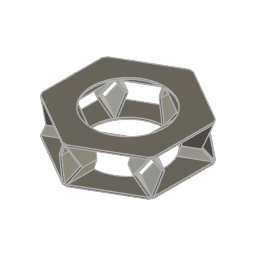
Parametric TPU Printable Horn Ring Support (Autodesk Fusion 360 design; units mm, degrees)
Autodesk Fusion 360 part; units mm, degrees
sketch "Sketch1" plane through (0, 0, 0) normal (1, 0, 0) x (0, 1, 0) in component "Component"
  line L0 (0, 0) -> (35, 0)
  line L1 (35, 9) -> (20, 9)
  line L2 (35, 9) -> (35, 10)
  line L3 (35, 10) -> (20, 10)
  line L4 (20, 10) -> (20, 9)
  line L5 (20, 9) -> (23.5, 0)
  line L6 (35, 9) -> (31.5, 0)
  line L7 (23.5, 0) -> (31.5, 0)
  line L8 (35, 9) -> (35, 0)
  line L9 (20, 9) -> (20, 0)
  dimension "d27" = 35
  dimension "d28" = 20
  dimension "d29" = 1
  dimension "d30" = 10
  dimension "d34" = 8
  constraint coincident L0.start origin
  constraint horizontal L0
  constraint horizontal L1
  constraint perpendicular L1 L2
  constraint perpendicular L2 L3
  constraint perpendicular L3 L4
  constraint coincident L0 L5.end
  constraint coincident L0 L6.end
  constraint equal L5 L6
  constraint perpendicular L0 L8
  constraint coincident L0 L9.end
  constraint perpendicular L0 L9
  measures "d27" horizontal distance of L0.start L2.end
  measures "d28" horizontal distance of L0.start L3.end
  measures "d29" distance of L1.end L3.end
  measures "d30" vertical distance of L0.start L3.end
  measures "d34" distance of L5.end L6.end
sketch "Sketch2" plane through (0, 0, 0) normal (0, 1, 0) x (1, 0, 0) in component "Component"
  line L0 (0, -9) -> (5.1962, 0)
  line L1 (5.1962, 0) -> (6.3962, 0)
  line L2 (6.3962, 0) -> (1.2, -9)
  line L3 (1.2, -9) -> (0, -9)
  line L4 (0, 0) -> (0, -9) construction
  line L5 (0, 0) -> (0, -9) construction
  line L6 (-6.3962, 0) -> (-1.2, -9)
  line L7 (-5.1962, 0) -> (-6.3962, 0)
  line L8 (0, -9) -> (-5.1962, 0)
  line L9 (-1.2, -9) -> (0, -9)
  point P0 (0, -9)
  dimension "d35" = 1.2
  dimension "d36" = 60
  constraint coincident P0 L0.start
  constraint horizontal L1
  constraint parallel L0 L2
  constraint horizontal L3
  constraint coincident L4.start L5.start
  constraint symmetric P0 L4 L0.start
  constraint symmetric L0.end L4 L7.start
  constraint symmetric L1.end L4 L6.start
  constraint symmetric L2.end L4 L6.end
  constraint symmetric L5.start L4 origin
  constraint coincident L1 L4.start
  measures "d35" distance of L0.end L1.end
  measures "d36" angle of L0 L8
extrude "Extrude1" add sketch "Sketch2" along normal blind 15 from surface at 20 makes body 1 in component "Component"
extrude "Extrude2" cut sketch "Sketch1" along normal through all and the other way through all contours L0 L5 L9 | L0 L6 L8 bodies 1 in component "Component"
revolve "Revolve1" add sketch "Sketch1" angle 360 about axis through (0, 0, 1.75) along (0, 0, 1) separate body contours L1 L2 L3 L4 makes body 2 in component "Component"
sketch "Sketch3" plane through (0, 0, 10) normal (0, 0, 1) x (-1, 0, 0) in component "Component"
  circle A0 centre (0, 0) radius 20
  circle A1 centre (0, 0) radius 35
  line L0 (0, -35) -> (0, 0) construction
  circle A2 centre (0, 0) radius 20
  circle A3 centre (0, 0) radius 35
  line L1 (-1.2, -20) -> (-1.2, -35)
  line L2 (0, 0) -> (-30.3109, -17.5) construction
  line L3 (-29.6932, -18.5288) -> (-16.6894, -11.0211)
  line L4 (-16.6894, -11.0211) -> (-1.2, -20)
  line L5 (-29.6932, -18.5288) -> (-1.2, -35)
  point P0 (-1.2, -35)
  point P1 (0, -35)
  dimension "d56" = 60
  dimension "d57" = 1.2
  dimension "d58" = 1.2
  constraint coincident P1 L0.start
  constraint coincident A0.centre A1.centre
  constraint coincident A3 L2.end
  constraint coincident A3 L3.start
  constraint coincident A2 L3.end
  constraint parallel L2 L3
  constraint coincident L1.start L4.end
  constraint coincident P0 L1.end
  measures "d56" angle of L0 L2
  measures "d57" distance of P0 P1
  measures "d58" distance of L2.end L3.start
extrude "Extrude4" cut sketch "Sketch3" against normal up to surface (1 mm away) contours A1 A3 L5 bodies 2 in component "Component"
pattern_circular "C-Pattern2" count 6 over 360 about axis through (0, 0, 1.75) along (0, 0, 1) of "Extrude4" in component "Component"
pattern_circular "C-Pattern1" count 6 over 360 about axis through (0, 0, 1.75) along (0, 0, 1) of bodies 1 makes body 3 at (-21.195, 15.6226, 6) makes body 4 at (-24.127, -10.5441, 6) makes body 5 at (-2.9321, -26.1667, 6) makes body 6 at (26.4364, -11.8774, 6) makes body 7 at (21.195, 15.6226, 6) in component "Component"
combine "Combine1" operation add target body 1 tool bodies 7 6 5 3 4 2 in component "Component"
mirror "Mirror2" about plane through (0, 0, 0) normal (0, 0, 1) of bodies 1 merged in component "Component"
extrude "Extrude5" add sketch "Sketch3" along normal blind 0.2 from surface at -1 contours A0 A2 L4 picked at (-11.0178, -14.7006) bodies 1 in component "Component"
pattern_circular "C-Pattern4" count 6 over 360 about axis through (0, 0, 1.75) along (0, 0, 1) of "Extrude5" in component "Component"
component "Component" placed x (1, 0, 0) y (0, 1, 0) z (0, 0, 1) at (0, 0, 0)
equation "BearingOD = 70 mm"
equation "BearingID = 40 mm"
equation "BearingHeight = 20 mm"
equation "TopBottomThickness = 1 mm"
equation "SupportCount = 6"
equation "d27 = BearingOD / 2"
equation "d28 = BearingID / 2"
equation "d29 = TopBottomThickness"
equation "d30 = BearingHeight / 2"
equation "d35 = WallThickness"
equation "d37 = BearingID / 2"
equation "d38 = ( BearingOD - BearingID ) / 2"
equation "d42 = SupportCount"
equation "NozzleSize = 0.4 mm"
equation "WallThickness = 3 * NozzleSize"
equation "d56 = ( 360 / SupportCount ) * 1 deg"
equation "d58 = d57"
equation "LayerHeightForBridgyBit = 0.2 mm"
equation "d63 = LayerHeightForBridgyBit"
named bodies: "Bearing", "TopRing"
